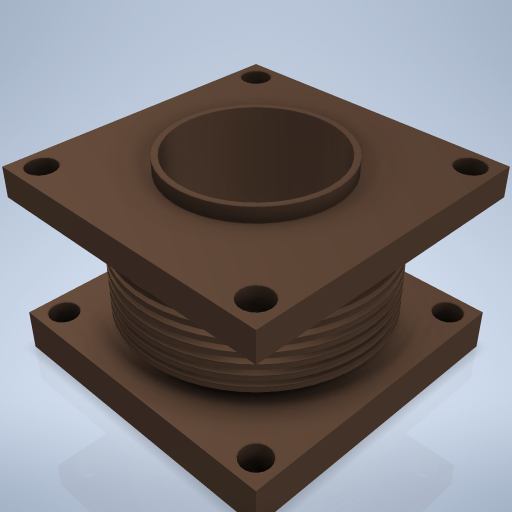
# Autodesk Inventor part: cylinder
Saved by Autodesk Inventor 2024.2 (Build 282272000, 272)
## iProperties
Created: 2024-05-14
Part Number: cylinder
Material: Bronze, Guss
Document SubType Name: Modeling
Designer: Fabri
Density: 8.87 g/cm^3
Appearance: Bronze - satiniert
Author: Fabri
Autodesk Inventor part; units mm, degrees
sketch "Skizze2" plane through (0, 0, 0) normal (0, 1, 0) x (-1, 0, 0)
  line L0 (0, 0) -> (14.5, 0)
  line L1 (14.5, 0) -> (14.5, -35.5)
  line L2 (14.5, -35.5) -> (0, -35.5)
  line L3 (0, -35.5) -> (0, 0)
  dimension "d2" = 29
  dimension "d3" = 35.5
  constraints: 8 end point, 3 perpendicular, 1 horizontal
  measures "d2" diameter of L1 L3
  measures "d3" distance between parallel lines of L2 L0
revolve "Umdrehung1" add sketch "Skizze2" angle 360 about axis through (0, 0, -35.5) along (0, 0, 1)
ref_plane "Arbeitsebene1" through (0, 0, 0) normal (1, 0, 0) x (0, 1, 0)
ref_plane "Arbeitsebene2" through (0, 0, -2.5) normal (0, 0, 1) x (1, 0, 0)
sketch "Skizze4" plane through (0, 0, -2.5) normal (0, 0, 1) x (1, 0, 0)
  line L0 (25, -25) -> (-25, -25)
  line L1 (-25, -25) -> (-25, 25)
  line L2 (-25, 25) -> (25, 25)
  line L3 (25, 25) -> (25, -25)
  line L4 (25, -25) -> (-25, 25) construction
  line L5 (-25, -25) -> (25, 25) construction
  point P0 (0, 0)
  dimension "d7" = 50
  dimension "d8" = 50
  constraints: 12 end point, 2 midpoint, 2 parallel, 1 horizontal, 1 perpendicular
  measures "d7" distance of L1.end L2.end
  measures "d8" distance of L0.end L1.end
extrude "Extrusion1" add sketch "Skizze4" against normal blind 5
ref_plane "Arbeitsebene3" through (0, 0, 0) normal (0, 1, 0) x (-1, 0, 0)
sketch "Skizze5" plane through (0, 0, 0) normal (0, 1, 0) x (-1, 0, 0)
  line L0 (14.5, -2.5) -> (14.5, 0) projected
  line L1 (14.5, -35.5) -> (14.5, -7.5) projected
  line L2 (14.5, -9.5) -> (22, -9.5)
  line L3 (22, -9.5) -> (22, -10.5)
  line L4 (22, -10.5) -> (14.5, -10.5)
  line L5 (25, -2.5) -> (-25, -2.5) projected
  line L6 (25, -2.5) -> (25, -7.5) projected
  line L7 (-25, -7.5) -> (25, -7.5) projected
  line L8 (-25, -2.5) -> (-25, -7.5) projected
  line L9 (0, 0) -> (0, -35.5)
  line L10 (14.5, -9.5) -> (14.5, -10.5)
  line L11 (14.5, -11.5) -> (22, -11.5)
  line L12 (22, -11.5) -> (22, -12.5)
  line L13 (22, -12.5) -> (14.5, -12.5)
  line L14 (14.5, -11.5) -> (14.5, -12.5)
  line L15 (14.5, -13.5) -> (22, -13.5)
  line L16 (22, -13.5) -> (22, -14.5)
  line L17 (22, -14.5) -> (14.5, -14.5)
  line L18 (14.5, -13.5) -> (14.5, -14.5)
  line L19 (14.5, -15.5) -> (22, -15.5)
  line L20 (22, -15.5) -> (22, -16.5)
  line L21 (22, -16.5) -> (14.5, -16.5)
  line L22 (14.5, -15.5) -> (14.5, -16.5)
  line L23 (14.5, -17.5) -> (22, -17.5)
  line L24 (22, -17.5) -> (22, -18.5)
  line L25 (22, -18.5) -> (14.5, -18.5)
  line L26 (14.5, -17.5) -> (14.5, -18.5)
  line L27 (14.5, -19.5) -> (22, -19.5)
  line L28 (22, -19.5) -> (22, -20.5)
  line L29 (22, -20.5) -> (14.5, -20.5)
  line L30 (14.5, -19.5) -> (14.5, -20.5)
  line L31 (14.5, -21.5) -> (22, -21.5)
  line L32 (22, -21.5) -> (22, -22.5)
  line L33 (22, -22.5) -> (14.5, -22.5)
  line L34 (14.5, -21.5) -> (14.5, -22.5)
  line L35 (14.5, -23.5) -> (22, -23.5)
  line L36 (22, -23.5) -> (22, -24.5)
  line L37 (22, -24.5) -> (14.5, -24.5)
  line L38 (14.5, -23.5) -> (14.5, -24.5)
  point P0 (22, -10)
  point P1 (18.25, -13.5)
  point P2 (18.25, -22.5)
  dimension "d12" = 1
  dimension "d13" = 2
  dimension "d14" = 44
  dimension "d15" = 1
  dimension "d16" = 1
  dimension "d17" = 1
  dimension "d18" = 1
  dimension "d19" = 1
  dimension "d20" = 1
  dimension "d21" = 1
  dimension "d22" = 1
  dimension "d23" = 1
  dimension "d24" = 1
  dimension "d25" = 1
  dimension "d26" = 1
  dimension "d27" = 1
  dimension "d28" = 1
  dimension "d29" = 44
  constraints: 66 end point, 12 horizontal, 10 point on line, 9 vertical, 7 perpendicular, 3 midpoint, 1 vertical alignment, 17 other
  measures "d12" distance between parallel lines of L4 L2
  measures "d13" distance between parallel lines of L2 L7
  measures "d14" diameter of point (22, -10) L9
  measures "d15" distance between parallel lines of L13 L11
  measures "d16" distance between parallel lines of L17 L15
  measures "d17" distance between parallel lines of L21 L19
  measures "d18" distance between parallel lines of L25 L23
  measures "d19" distance between parallel lines of L11 L4
  measures "d20" distance from line of point (18.25, -13.5) L13
  measures "d21" distance between parallel lines of L19 L17
  measures "d22" distance between parallel lines of L23 L21
  measures "d23" distance between parallel lines of L29 L27
  measures "d24" distance between parallel lines of L33 L31
  measures "d25" distance between parallel lines of L37 L35
  measures "d26" distance between parallel lines of L27 L25
  measures "d27" distance between parallel lines of L31 L29
  measures "d28" distance from line of L35 point (18.25, -22.5)
  measures "d29" diameter of L12 L9
revolve "Umdrehung2" add sketch "Skizze5" angle 360 about axis through (0, 0, 0) along (0, 0, -1) contours L1 L2 L3 L4 | L1 L11 L12 L13 | L1 L15 L16 L17 | L1 L19 L20 L21 | L1 L23 L24 L25 | L1 L27 L28 L29 | L1 L31 L32 L33 | L1 L35 L36 L37
ref_plane "Arbeitsebene4" through (0, 0, -35.5) normal (0, 0, -1) x (-1, 0, 0)
sketch "Skizze6" plane through (0, 0, -35.5) normal (0, 0, -1) x (-1, 0, 0)
  line L0 (-25, 25) -> (25, 25)
  line L1 (25, 25) -> (25, -25)
  line L2 (25, -25) -> (-25, -25)
  line L3 (-25, -25) -> (-25, 25)
  line L4 (-25, 25) -> (25, -25) construction
  line L5 (25, 25) -> (-25, -25) construction
  point P0 (0, 0)
  dimension "d32" = 50
  dimension "d33" = 50
  constraints: 12 end point, 2 midpoint, 2 parallel, 1 horizontal, 1 perpendicular
  measures "d32" distance of L1.end L2.end
  measures "d33" distance of L0.end L1.end
extrude "Extrusion2" add sketch "Skizze6" against normal blind 7
sketch "Skizze7" plane through (25, -25, -35.5) normal (0, 0, -1) x (-1, 0, 0)
  point P0 (25, 25)
  point P1 (25, 25)
  constraints: 1 coincident
hole "Bohrung1" at (0, 0, -35.5) direction (0, 0, 1) diameter 27 depth 35.5
sketch "Skizze8" plane through (25, -25, -35.5) normal (0, 0, -1) x (-1, 0, 0)
  line L0 (0, 0) -> (50, 0) projected
  line L1 (25, 0) -> (25, 50) construction
  line L2 (50, 50) -> (0, 50) projected
  line L3 (50, 50) -> (50, 0) projected
  line L4 (50, 25) -> (0, 25) construction
  line L5 (0, 0) -> (0, 50) projected
  point P0 (25, 25)
  point P1 (46.124, 3.876)
  point P2 (3.876, 3.876)
  point P3 (46.124, 46.124)
  point P4 (3.876, 46.124)
  dimension "d75" = 42.248
  dimension "d76" = 42.248
  constraints: 4 end point, 4 midpoint, 2 horizontal alignment, 2 symmetric about line, 2 vertical alignment
  measures "d75" distance of point (46.124, 46.124) point (46.124, 3.876)
  measures "d76" distance of point (3.876, 46.124) point (46.124, 46.124)
hole "Bohrung2" at (-21.124, -21.124, -35.5) at (21.124, -21.124, -35.5) at (-21.124, 21.124, -35.5) at (21.124, 21.124, -35.5) direction (0, 0, 1) diameter 5 depth 7
sketch "Skizze9" plane through (0, 0, -2.5) normal (0, 0, 1) x (1, 0, 0)
  line L0 (25, 25) -> (25, -25) projected
  line L1 (25, 0) -> (-25, 0) construction
  line L2 (-25, -25) -> (-25, 25) projected
  line L3 (-25, 25) -> (25, 25) projected
  line L4 (0, 25) -> (0, -36.4207) construction
  point P0 (0, 0)
  point P1 (-21.124, 21.124)
  point P2 (21.124, 21.124)
  point P3 (-21.124, -21.124)
  point P4 (21.124, -21.124)
  dimension "d73" = 42.248
  dimension "d74" = 42.248
  constraints: 4 end point, 3 midpoint, 3 symmetric about line, 2 horizontal alignment, 1 vertical
  measures "d73" distance of point (-21.124, 21.124) point (21.124, 21.124)
  measures "d74" distance of point (-21.124, -21.124) point (-21.124, 21.124)
hole "Bohrung3" at (-21.124, 21.124, -2.5) at (21.124, 21.124, -2.5) at (-21.124, -21.124, -2.5) at (21.124, -21.124, -2.5) direction (0, 0, -1) diameter 5 depth 5
equation "\"d16\" = d15"
equation "\"d17\" = d15"
equation "\"d18\" = d15"
equation "\"d26\" = d22"
equation "\"d27\" = d22"
equation "\"d28\" = d22"
equation "\"d76\" = d75"
equation "\"d74\" = d73"
